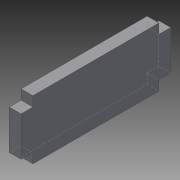
# Autodesk Inventor part: Mid rib support
Saved by Autodesk Inventor 2015 (Build 190159000, 159)
## iProperties
Created: 2014-11-13
Part Number: Mid rib support
Material: Generic
Document SubType Name: Modeling
Designer: karl
Density: 1 g/cm^3
Appearance: Default
Author: karl
Autodesk Inventor part; units mm, degrees
ref_plane "YZ Plane" through (0, 0, 0) normal (1, 0, 0) x (0, 1, 0)
ref_plane "XZ Plane" through (0, 0, 0) normal (0, 1, 0) x (-1, 0, 0)
ref_plane "XY Plane" through (0, 0, 0) normal (0, 0, 1) x (1, 0, 0)
sketch "Sketch1" plane through (0, 0, 0) normal (1, 0, 0) x (0, 1, 0)
  line L0 (-16, -7.5) -> (16, -7.5)
  line L1 (16, -7.5) -> (16, 7.5)
  line L2 (16, 7.5) -> (-16, 7.5)
  line L3 (-16, 7.5) -> (-16, -7.5)
  line L4 (-16, -7.5) -> (16, 7.5) construction
  line L5 (16, -7.5) -> (-16, 7.5) construction
  point P0 (0, 0)
  dimension "d0" = 32
  dimension "d1" = 15
  constraints: 12 end point, 2 midpoint, 2 parallel, 1 horizontal, 1 perpendicular
  measures "d0" distance of L2.end L1.end
  measures "d1" distance of L1.end L0.end
extrude "Extrusion1" add sketch "Sketch1" along normal blind 3
sketch "Sketch2" plane through (3, 0, 0) normal (1, 0, 0) x (0, 0, -1)
  line L0 (7.5, 16) -> (-7.5, 16) projected
  line L1 (-5, 16) -> (5, 16)
  line L2 (5, 16) -> (5, 19)
  line L3 (5, 19) -> (-5, 19)
  line L4 (-5, 19) -> (-5, 16)
  line L5 (-5, -16) -> (5, -16)
  line L6 (5, -16) -> (5, -19)
  line L7 (5, -19) -> (-5, -19)
  line L8 (-5, -19) -> (-5, -16)
  line L9 (-7.5, -16) -> (7.5, -16) projected
  point P0 (0, 0)
  point P1 (0, 19)
  dimension "d4" = 10
  dimension "d5" = 3
  dimension "d6" = 10
  dimension "d7" = 3
  constraints: 16 end point, 4 parallel, 2 horizontal, 2 perpendicular, 2 point on line, 1 collinear, 1 midpoint, 1 vertical alignment
  measures "d4" distance of L3.end L2.end
  measures "d5" distance of L2.end L1.end
  measures "d6" distance of L6.end L7.end
  measures "d7" distance of L5.end L6.end
extrude "Extrusion2" add sketch "Sketch2" against normal blind 3
body "Solid1"
